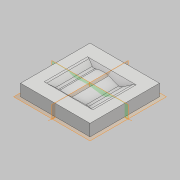
# Autodesk Inventor part: Placa - Abrasión punto Silla
Saved by Autodesk Inventor 2017 (Build 210142000, 142)
## iProperties
Part Number: Placa - Abrasión punto Silla
Material: Genérico
Document SubType Name: Modeling
Designer: franc
Density: 1 g/cm^3
Appearance: Valor por defecto
Author: franc
Autodesk Inventor part; units mm, degrees
sketch "Boceto1" plane through (0, 0, 0) normal (0, 0, 1) x (1, 0, 0)
  line L0 (-75, 75) -> (75, 75)
  line L1 (75, 75) -> (75, -75)
  line L2 (75, -75) -> (-75, -75)
  line L3 (-75, -75) -> (-75, 75)
  line L4 (-75, 75) -> (75, -75) construction
  line L5 (75, 75) -> (-75, -75) construction
  point P0 (0, 0)
  dimension "d0" = 150
  dimension "d1" = 150
  constraints: 12 end point, 2 midpoint, 2 parallel, 1 horizontal, 1 perpendicular
  measures "d0" distance of L1.end L2.end
  measures "d1" distance of L0.end L1.end
extrude "Extrusión1" add sketch "Boceto1" along normal blind 25.4
sketch "Boceto2" plane through (0, 0, 0) normal (0, 1, 0) x (-1, 0, 0)
  line L0 (-75, 25.4) -> (75, 25.4) projected
  line L1 (0, 25.4) -> (-45.0693, 25.4)
  line L2 (-45.0693, 25.4) -> (-30.9272, 25.4) construction
  line L3 (-30.4041, 15.4) -> (12.482, 21.4)
  line L4 (12.482, 21.4) -> (32.0178, 18.4)
  line L5 (0, 25.4) -> (45.9037, 25.4)
  line L6 (-30.4041, 15.4) -> (-50, 25.4)
  line L7 (-45.0693, 25.4) -> (-50, 25.4)
  line L8 (-75, 0) -> (-75, 25.4) projected
  line L9 (32.0178, 18.4) -> (50, 25.4)
  line L10 (50, 25.4) -> (45.9037, 25.4)
  line L11 (75, 0) -> (75, 25.4) projected
  point P0 (0, 0)
  dimension "d33" = 4
  dimension "d34" = 7
  dimension "d35" = 10
  dimension "d36" = 22
  dimension "d41" = 150
  dimension "d42" = 145
  dimension "d45" = 100
  dimension "d46" = 25
  dimension "d47" = 25
  constraints: 18 end point, 4 point on line, 1 collinear, 1 horizontal, 1 midpoint
  measures "d33" distance from line of L0 L3.end
  measures "d34" distance from line of L0 L4.end
  measures "d35" distance from line of L0 L3.start
  measures "d36" distance of L3.start L6.end
  measures "d41" angle of L4 L9
  measures "d42" angle of L3 L6
  measures "d45" distance of L6.end L9.end
  measures "d46" distance from line of L8 L6.end
  measures "d47" distance from line of L11 L9.end
extrude "Extrusión2" cut sketch "Boceto2" along normal blind 35
fillet "Empalme2" radius 90 1 edges at (-12.482, 17.5, 21.4)
chamfer "Chaflán1" distance 9.85 angle 50 1 edges at (0, 35, 25.4)
mirror "Simetría1" about plane through (0, 0, 0) normal (0, 1, 0) of "Extrusión2", "Empalme2", "Chaflán1"
fillet "Empalme15" radius 12 2 edges at (-32.0178, 0, 18.4) (30.4041, 0, 15.4)
fillet "Empalme16" radius 12 2 edges at (-50, 0, 25.4) (50, 0, 25.4)
